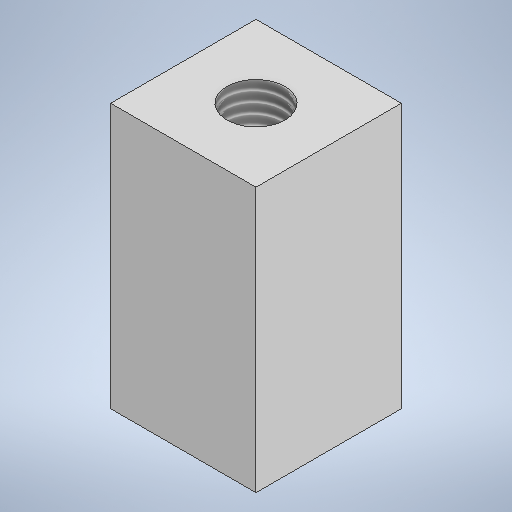
# Autodesk Inventor part: Rb PEEK - Soporte
Saved by Autodesk Inventor 2025.3 (Build 293356000, 356)
## iProperties
Created: 2025-05-09
Part Number: Rb PEEK - Soporte
Material: Generic
Document SubType Name: Modeling
Designer: E. Moreno
Density: 1 g/cm^3
Appearance: Default
Title: Rb PEEK - Soporte
Author: E. Moreno
Autodesk Inventor part; units mm, degrees
ref_plane "YZ Plane" through (0, 0, 0) normal (1, 0, 0) x (0, 1, 0)
ref_plane "XZ Plane" through (0, 0, 0) normal (0, 1, 0) x (-1, 0, 0)
ref_plane "XY Plane" through (0, 0, 0) normal (0, 0, 1) x (1, 0, 0)
sketch "Sketch1" plane through (0, 0, 0) normal (1, 0, 0) x (0, 1, 0)
  line L0 (-9.1, 5) -> (9.1, 5)
  line L1 (9.1, 5) -> (9.1, -5)
  line L2 (9.1, -5) -> (-9.1, -5)
  line L3 (-9.1, -5) -> (-9.1, 5)
  line L4 (-9.1, 5) -> (9.1, -5) construction
  line L5 (9.1, 5) -> (-9.1, -5) construction
  point P0 (0, 0)
  dimension "d0" = 18.2
  dimension "d1" = 10
  constraints: 12 end point, 2 midpoint, 2 parallel, 1 horizontal, 1 perpendicular
  measures "d0" distance of L1.end L2.end
  measures "d1" distance of L0.end L1.end
extrude "Extrusion1" add sketch "Sketch1" along normal blind 10
sketch "Sketch2" plane through (0, 9.1, 5) normal (0, 1, 0) x (1, 0, 0)
  line L0 (0, 5) -> (5, 5)
  circle A0 centre (5, 5) radius 2
  dimension "d4" = 5
  dimension "d5" = 4
  constraints: 2 end point, 1 centre point, 1 coincident, 1 horizontal
  measures "d4" distance of L0.start L0.end
  measures "d5" diameter of A0
extrude "Extrusion2" cut sketch "Sketch2" against normal blind 8
thread "Thread1" size "M4x0.7" class "6H" standard "ANSI Metric M Profile" full length
sketch "Sketch3" plane through (0, -9.1, -5) normal (0, -1, 0) x (1, 0, 0)
  line L0 (0, 5) -> (5, 5)
  circle A0 centre (5, 5) radius 2
  dimension "d10" = 5
  dimension "d11" = 4
  constraints: 2 end point, 1 centre point, 1 coincident, 1 horizontal
  measures "d10" distance of L0.start L0.end
  measures "d11" diameter of A0
extrude "Extrusion3" cut sketch "Sketch3" against normal blind 8
thread "Thread2" size "M4x0.7" class "6H" standard "ANSI Metric M Profile" full length
body "Solid1"
